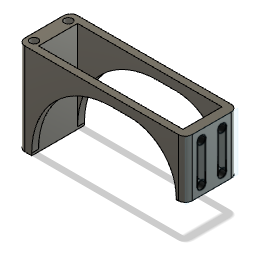
upper sensor arm v1 (Autodesk Fusion 360 design; units mm, degrees)
Autodesk Fusion 360 part; units mm, degrees
sketch "Sketch1" plane through (0, 0, 0) normal (0, 1, 0) x (1, 0, 0)
  circle A0 centre (0, 0) radius 1.75
  circle A1 centre (0, 15) radius 1.75
  line L0 (-3, 19) -> (3, 19)
  line L1 (3, 19) -> (3, -4)
  line L2 (3, -4) -> (-3, -4)
  line L3 (-3, -4) -> (-3, 19)
  dimension "d1" = 3.5
  dimension "d2" = 3.5
  dimension "d3" = 15
  dimension "d4" = 4
  dimension "d5" = 4
  constraint coincident A0.centre origin
  constraint horizontal L0
  constraint vertical L1
  constraint horizontal L2
  constraint vertical L3
  constraint vertical A0.centre A1.centre
  measures "d1" diameter of A0
  measures "d2" diameter of A1
  measures "d3" distance of A0.centre A1.centre
  measures "d4" distance of A0.centre L2
  measures "d5" distance of A1.centre L0
extrude "Extrude1" add sketch "Sketch1" along normal blind 40 makes body 1
sketch "Sketch2" plane through (0, 40, 0) normal (0, 1, 0) x (-1, 0, 0)
  circle A0 centre (0, -15) radius 1.75
  circle A1 centre (0, 0) radius 1.75
  line L0 (3, 4) -> (-3, 4)
  line L1 (-3, 4) -> (-3, -19)
  line L2 (-3, -19) -> (3, -19)
  line L3 (3, -19) -> (3, 4)
  line L4 (-66, -19) -> (-70, -19)
  line L5 (-70, -19) -> (-70, 4)
  line L6 (-70, 4) -> (-66, 4)
  line L7 (-66, 4) -> (-66, -19)
  dimension "d8" = 4
  dimension "d10" = 70
  constraint horizontal L4
  constraint vertical L5
  constraint horizontal L6
  constraint vertical L7
  constraint horizontal L1.end L4.start
  constraint horizontal L0.end L6.end
  measures "d8" distance of L4.start L4.end
  measures "d10" distance of A1.centre L5
extrude "Extrude2" add sketch "Sketch2" against normal blind 25 separate body contours L4 L5 L6 L7 makes body 2
sketch "Sketch3" plane through (0, 40, 0) normal (0, 1, 0) x (-1, 0, 0)
  circle A0 centre (0, -15) radius 1.75
  circle A1 centre (0, 0) radius 1.75
  line L0 (3, 4) -> (-3, 4)
  line L1 (-3, 4) -> (-3, -19)
  line L2 (-3, -19) -> (3, -19)
  line L3 (3, -19) -> (3, 4)
  line L4 (-3, -19) -> (-66, -19)
  line L5 (-66, -19) -> (-66, -16)
  line L6 (-66, -16) -> (-3, -16)
  line L7 (-3, -16) -> (-3, -19)
  line L8 (-3, 4) -> (-66, 4)
  line L9 (-66, 4) -> (-66, 1)
  line L10 (-66, 1) -> (-3, 1)
  line L11 (-3, 1) -> (-3, 4)
  constraint horizontal L4
  constraint vertical L5
  constraint horizontal L6
  constraint vertical L7
  constraint coincident L1.end L2.start
  constraint horizontal L8
  constraint vertical L9
  constraint horizontal L10
  constraint vertical L11
  constraint coincident L0.end L1.start
extrude "Extrude3" add sketch "Sketch3" against normal blind 4 contours L1 L8 L9 L10 L11 | L1 L4 L5 L6 L7 bodies 1 2
fillet "Fillet1" radius 20 2 edges at (66, 36, -17.5) (66, 36, 2.5) on bodies 1
fillet "Fillet2" radius 35 2 edges at (3, 36, -17.5) (3, 36, 2.5) on bodies 1
sketch "Sketch4" plane through (70, 0, 0) normal (1, 0, 0) x (0, 0, -1)
  line L0 (19, 40) -> (-4, 40)
  line L1 (-4, 40) -> (-4, 15)
  line L2 (-4, 15) -> (19, 15)
  line L3 (19, 15) -> (19, 40)
  circle A0 centre (3, 36) radius 1.75
  circle A1 centre (3, 19) radius 1.75
  circle A2 centre (12, 36) radius 1.75
  circle A3 centre (12, 19) radius 1.75
  line L4 (4.75, 19) -> (4.75, 36)
  line L5 (1.25, 36) -> (1.25, 19)
  line L6 (13.75, 36) -> (13.75, 19)
  line L7 (10.25, 19) -> (10.25, 36)
  dimension "d17" = 3.5
  dimension "d18" = 3.5
  dimension "d19" = 3.5
  dimension "d20" = 3.5
  dimension "d21" = 7
  dimension "d22" = 7
  dimension "d23" = 4
  dimension "d24" = 4
  constraint vertical A2.centre A3.centre
  constraint vertical A0.centre A1.centre
  constraint horizontal A0.centre A2.centre
  constraint horizontal A1.centre A3.centre
  constraint coincident A1 L4.start
  constraint coincident A0 L4.end
  constraint tangent A0 L4
  constraint coincident A0 L5.start
  constraint coincident A1 L5.end
  constraint tangent A0 L5
  constraint tangent A1 L5
  constraint tangent A1 L4
  constraint coincident A2 L6.start
  constraint coincident A3 L6.end
  constraint tangent A3 L6
  constraint coincident A3 L7.start
  constraint coincident A2 L7.end
  constraint tangent A2 L7
  constraint tangent A3 L7
  constraint tangent A2 L6
  measures "d17" diameter of A0
  measures "d18" diameter of A1
  measures "d19" diameter of A2
  measures "d20" diameter of A3
  measures "d21" distance of L3 A2.centre
  measures "d22" distance of L1 A0.centre
  measures "d23" distance of L0 A0.centre
  measures "d24" distance of L2 A1.centre
extrude "Extrude4" cut sketch "Sketch4" against normal up to surface (4 mm away) contours A0 | A0 A1 L4 L5 | A1 | A2 | A2 A3 L6 L7 | A3 bodies 1
fillet "Fillet3" radius 3 4 edges at (-3, 20, -19) (-3, 20, 4) (70, 27.5, -19) (70, 27.5, 4) on bodies 1
equation "d21 = d22"
equation "d24 = d23"
